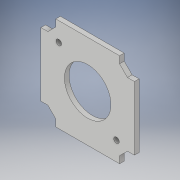
# Autodesk Inventor part: LC_sample_holder_insert
Saved by Autodesk Inventor 2019 (Build 230136000, 136)
## iProperties
Created: 2021-05-27
Part Number: LC_sample_holder_insert
Material: Generic
Document SubType Name: Modeling
Designer: marsikovabarbora
Density: 1 g/cm^3
Appearance: Default
Author: marsikovabarbora
Autodesk Inventor part; units mm, degrees
ref_plane "YZ Plane" through (0, 0, 0) normal (1, 0, 0) x (0, 1, 0)
ref_plane "XZ Plane" through (0, 0, 0) normal (0, 1, 0) x (-1, 0, 0)
ref_plane "XY Plane" through (0, 0, 0) normal (0, 0, 1) x (1, 0, 0)
sketch "Sketch1" plane through (0, 0, 0) normal (0, 0, 1) x (1, 0, 0)
  line L0 (-38.1609, 0) -> (53.0268, 0) construction
  line L1 (0, -35.8177) -> (0, 38.9679) construction
  line L2 (0, 0) -> (28.2843, 28.2843) construction
  line L3 (0, 0) -> (40, 0) construction
  line L4 (0, 24.9041) -> (16.9, 24.9041)
  line L5 (16.9, 24.9041) -> (16.9, 21.2841)
  line L6 (16.9, 21.2841) -> (19.092, 19.092)
  line L7 (24.9041, 0) -> (24.9041, 16.9)
  line L8 (24.9041, 16.9) -> (21.2841, 16.9)
  line L9 (21.2841, 16.9) -> (19.092, 19.092)
  line L10 (0, 24.9041) -> (-16.9, 24.9041)
  line L11 (-16.9, 24.9041) -> (-16.9, 21.2841)
  line L12 (-16.9, 21.2841) -> (-19.092, 19.092)
  line L13 (-24.9041, 0) -> (-24.9041, 16.9)
  line L14 (-24.9041, 16.9) -> (-21.2841, 16.9)
  line L15 (-21.2841, 16.9) -> (-19.092, 19.092)
  line L16 (0, -24.9041) -> (16.9, -24.9041)
  line L17 (16.9, -24.9041) -> (16.9, -21.2841)
  line L18 (16.9, -21.2841) -> (19.092, -19.092)
  line L19 (24.9041, 0) -> (24.9041, -16.9)
  line L20 (24.9041, -16.9) -> (21.2841, -16.9)
  line L21 (21.2841, -16.9) -> (19.092, -19.092)
  line L22 (0, -24.9041) -> (-16.9, -24.9041)
  line L23 (-16.9, -24.9041) -> (-16.9, -21.2841)
  line L24 (-16.9, -21.2841) -> (-19.092, -19.092)
  line L25 (-24.9041, 0) -> (-24.9041, -16.9)
  line L26 (-24.9041, -16.9) -> (-21.2841, -16.9)
  line L27 (-21.2841, -16.9) -> (-19.092, -19.092)
  circle A0 centre (0, 0) radius 12.5
  circle A1 centre (-15.5, 15) radius 1.5
  line L28 (-18.5, 18) -> (-12.5, 18) construction
  line L29 (-12.5, 18) -> (-12.5, -12) construction
  line L30 (-12.5, -12) -> (-18.5, -12) construction
  line L31 (-18.5, -12) -> (-18.5, 18) construction
  line L32 (-15.5, 18) -> (-15.5, -12) construction
  circle A2 centre (15.5, -15) radius 1.5
  line L33 (-17.13, 25.1341) -> (0, 25.1341)
  line L34 (0, 25.1341) -> (17.13, 25.1341)
  line L35 (17.13, 25.1341) -> (17.13, 21.3793)
  line L36 (17.13, 21.3793) -> (19.2547, 19.2547)
  line L37 (19.2547, 19.2547) -> (21.3793, 17.13)
  line L38 (21.3793, 17.13) -> (25.1341, 17.13)
  line L39 (25.1341, 17.13) -> (25.1341, 0)
  line L40 (25.1341, 0) -> (25.1341, -17.13)
  line L41 (25.1341, -17.13) -> (21.3793, -17.13)
  line L42 (21.3793, -17.13) -> (19.2547, -19.2547)
  line L43 (19.2547, -19.2547) -> (17.13, -21.3793)
  line L44 (17.13, -21.3793) -> (17.13, -25.1341)
  line L45 (17.13, -25.1341) -> (0, -25.1341)
  line L46 (0, -25.1341) -> (-17.13, -25.1341)
  line L47 (-17.13, -25.1341) -> (-17.13, -21.3793)
  line L48 (-17.13, -21.3793) -> (-19.2547, -19.2547)
  line L49 (-19.2547, -19.2547) -> (-21.3793, -17.13)
  line L50 (-21.3793, -17.13) -> (-25.1341, -17.13)
  line L51 (-25.1341, -17.13) -> (-25.1341, 0)
  line L52 (-25.1341, 0) -> (-25.1341, 17.13)
  line L53 (-25.1341, 17.13) -> (-21.3793, 17.13)
  line L54 (-21.3793, 17.13) -> (-19.2547, 19.2547)
  line L55 (-19.2547, 19.2547) -> (-17.13, 21.3793)
  line L56 (-17.13, 21.3793) -> (-17.13, 25.1341)
  dimension "d0" = 45
  dimension "d1" = 16.9
  dimension "d2" = 3.62
  dimension "d3" = 3.1
  dimension "d4" = 25
  dimension "d5" = 3
  dimension "d11" = 6
  dimension "d12" = 3
  dimension "d14" = 15
  dimension "d15" = 3
  dimension "d16" = 15
  dimension "d17" = 15.5
  dimension "d18" = 15.5
  dimension "d19" = 30
  dimension "d20" = 0.23
  constraints: 110 end point, 20 symmetric about line, 4 perpendicular, 3 centre point, 3 horizontal, 3 point on line, 2 midpoint, 2 parallel, 1 coincident, 1 equal length, 1 tangent, 23 other
  measures "d0" angle of L3 L2
  measures "d1" distance of L4.start L4.end
  measures "d2" distance of L4.end L5.end
  measures "d3" distance of L5.end L6.end
  measures "d4" diameter of A0
  measures "d5" diameter of A1
  measures "d11" distance of L28.start L28.end
  measures "d12" distance from line of L28 A1.centre
  measures "d14" distance from line of L0 A1.centre
  measures "d15" diameter of A2
  measures "d16" distance from line of L0 A2.centre
  measures "d17" distance from line of L1 A2.centre
  measures "d18" distance from line of L1 A1.centre
  measures "d19" distance of L30.end L28.start
  measures "d20" distance between parallel lines of L10 L33
extrude "Extrusion1" add sketch "Sketch1" along normal blind 2.5 contours L4 L5 L6 L9 L8 L7 L19 L20 L21 L18 L17 L16 L22 L23 L24 L27 L26 L25 L13 L14 L15 L12 L11 L10 | L33 L34 L35 L36 L37 L38 L39 L40 L41 L42 L43 L44 L45 L46 L47 L48 L49 L50 L51 L52 L53 L54 L55 L56
body "Solid1"
